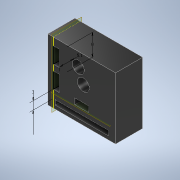
# Autodesk Inventor part: Pressuresensor_Holder
Saved by Autodesk Inventor 2022 (Build 260153000, 153)
## iProperties
Created: 2024-04-03
Part Number: Pressuresensor_Holder
Material: Generic
Document SubType Name: Modeling
Designer: Gotham City
Density: 1 g/cm^3
Appearance: Default
Comments: File was created by BTDwgCreate
Autodesk Inventor part; units mm, degrees
ref_plane "YZ Plane" through (0, 0, 0) normal (1, 0, 0) x (0, 1, 0)
ref_plane "XZ Plane" through (0, 0, 0) normal (0, 1, 0) x (-1, 0, 0)
ref_plane "XY Plane" through (0, 0, 0) normal (0, 0, 1) x (1, 0, 0)
sketch "Sketch1" plane through (0, 0, 0) normal (0, 0, 1) x (1, 0, 0)
  point P0 (0, 0)
sketch "MODELSKETCH_VISIBLE" plane through (0, 0, 0) normal (0, 0, 1) x (1, 0, 0)
  line L0 (12.5, 0) -> (12.5, 22.75)
  line L1 (-12.5, 0) -> (-12.5, 22.75)
  line L2 (-9.8, 1.3) -> (9.8, 1.3)
  line L3 (12.5, 0) -> (-12.5, 0)
  line L4 (-9.8, 3.05) -> (-9.8, 1.3)
  circle A0 centre (-1.3, 17.75) radius 2.2
  line L5 (9.8, 3.05) -> (9.8, 1.3)
  line L6 (-9.8, 3.05) -> (9.8, 3.05)
  line L7 (12.5, 22.75) -> (-12.5, 22.75)
  circle A1 centre (0.6, 12.99) radius 2.2
  constraints: 16 end point, 2 centre point
extrude "Extrusion1" add sketch "MODELSKETCH_VISIBLE" along normal blind 10
sketch "Sketch3" plane through (-9.8, 1.3, 0) normal (0, 1, 0) x (1, 0, 0)
  line L0 (19.6, 36.5) -> (0, 36.5)
  line L1 (0, 36.5) -> (0, -19)
  line L2 (0, -19) -> (19.6, -19)
  line L3 (19.6, -19) -> (19.6, 36.5)
  line L4 (19.6, -10) -> (0, -10) projected
  point P0 (9.8, 0)
  point P1 (19.6, 0)
  point P2 (0, 0)
  dimension "d2" = 55.5
  dimension "d3" = 9
  constraints: 8 end point, 2 parallel, 2 point on line, 1 horizontal, 1 perpendicular
  measures "d2" distance of L0.end L1.end
  measures "d3" distance between parallel lines of L2 L4
extrude "Extrusion2" add sketch "Sketch3" along normal blind 1.5 separate body
ref_plane "Work Plane1" through (-10.5, 0, 0) normal (-1, 0, 0) x (0, 0, 1)
sketch "Sketch4" plane through (-10.5, 0, 0) normal (-1, 0, 0) x (0, 0, 1)
  line L0 (2.45, 10.4667) -> (5, 11.939)
  line L1 (5, 11.939) -> (7.55, 10.4667) construction
  line L2 (7.55, 10.4667) -> (7.55, 7.5222) construction
  line L3 (7.55, 7.5222) -> (5, 6.05) construction
  line L4 (5, 6.05) -> (2.45, 7.5222)
  line L5 (2.45, 7.5222) -> (2.45, 10.4667)
  line L6 (5, 6.05) -> (10, 6.05)
  line L7 (10, 0) -> (10, 22.75) projected
  line L8 (5, 11.939) -> (10, 11.939)
  line L9 (10, 6.05) -> (10, 11.939)
  line L10 (0, 22.75) -> (10, 22.75) construction
  line L11 (5, 22.75) -> (5, 0) construction
  line L12 (0, 0) -> (10, 0) construction
  line L13 (0, 3.05) -> (10, 3.05) construction
  line L14 (0, 0) -> (0, 22.75) construction
  line L15 (0, 12.9945) -> (10, 12.9945) construction
  line L16 (2.45, 15.5222) -> (5, 14.05)
  line L17 (5, 14.05) -> (7.55, 15.5222) construction
  line L18 (7.55, 15.5222) -> (7.55, 18.4667) construction
  line L19 (7.55, 18.4667) -> (5, 19.939) construction
  line L20 (5, 19.939) -> (2.45, 18.4667)
  line L21 (2.45, 18.4667) -> (2.45, 15.5222)
  line L22 (5, 19.939) -> (10, 19.939)
  line L23 (5, 14.05) -> (10, 14.05)
  line L24 (10, 19.939) -> (10, 14.05)
  point P0 (5, 8.9945)
  point P1 (5, 16.9945)
  point P2 (10, 19.939)
  dimension "d7" = 5.1
  dimension "d14" = 3
  dimension "d40" = 8
  constraints: 40 end point, 9 symmetric about line, 5 point on line, 2 midpoint, 2 perpendicular, 1 horizontal, 1 parallel, 1 vertical, 13 other
  measures "d7" distance between parallel lines of L5 L2
  measures "d14" distance between parallel lines of L6 L13
  measures "d40" distance of point (5, 16.994) point (5, 8.994)
extrude "Extrusion3" cut sketch "Sketch4" against normal blind 2.2 bodies 1
sketch "Sketch5" plane through (-12.5, 0, 0) normal (-1, 0, 0) x (0, 0, 1)
  point P0 (0, 0)
  point P1 (5, 8.9945)
  point P2 (5, 16.9945)
hole "Hole2" at (-12.5, 8.9945, 5) at (-12.5, 16.9945, 5) direction (1, 0, 0) diameter 2.6 depth 7 tip angle 118 bodies 1 clearance for "Socket Head Cap Screw ISO 4762" size "M2.5" standard "ISO"
sketch "Sketch6" plane through (-12.5, 0, 0) normal (0, -1, 0) x (1, 0, 0)
  line L0 (25, 0) -> (25, 10) construction
  line L1 (25, 0) -> (0, 10) construction
  line L2 (0, 0) -> (0, 10) construction
  line L3 (25, 10) -> (0, 10) construction
  line L4 (0, 0) -> (25, 10) construction
  point P0 (12.5, 0)
  point P1 (12.5, 5)
  constraints: 4 end point, 1 coincident, 1 midpoint
hole "Hole3" at (0, 0, 5) direction (0, 1, 0) diameter 2.9 depth 8 tip angle 118 bodies 1 clearance for "Socket Head Cap Screw ISO 4762" size "M2.5" standard "ISO"
ref_plane "Work Plane2" through (-9.8, 5.05, 0) normal (0, -1, 0) x (1, 0, 0)
sketch "Sketch7" plane through (-9.8, 5.05, 0) normal (0, -1, 0) x (1, 0, 0)
  circle A0 centre (9.8, 5) radius 1.45 construction
  line L0 (7.25, 6.4722) -> (9.8, 7.9445) construction
  line L1 (9.8, 7.9445) -> (12.35, 6.4722) construction
  line L2 (12.35, 6.4722) -> (12.35, 3.5278)
  line L3 (12.35, 3.5278) -> (9.8, 2.0555)
  line L4 (9.8, 2.0555) -> (7.25, 3.5278)
  line L5 (7.25, 3.5278) -> (7.25, 6.4722)
  line L6 (12.35, 6.4722) -> (12.35, 10)
  line L7 (8.2, 10) -> (12.6, 10) projected
  line L8 (7.25, 6.4722) -> (7.25, 10)
  line L9 (19.6, 10) -> (0, 10) projected
  line L10 (7.25, 10) -> (12.35, 10)
  point P0 (9.8, 0)
  dimension "d37" = 5.1
  constraints: 18 end point, 2 point on line, 2 vertical, 1 coincident, 1 collinear, 1 parallel, 13 other
  measures "d37" distance between parallel lines of L5 L2
extrude "Extrusion4" cut sketch "Sketch7" against normal blind 2.2 bodies 1
sketch "Sketch8" plane through (0, 0, 0) normal (0, 0, -1) x (-1, 0, 0)
  circle A0 centre (1.3, 17.75) radius 2.2 projected
  line L0 (12.5, 18.2945) -> (12.5, 15.6945) projected
  point P0 (0, 0)
body "Solid1"
body "Solid2"
